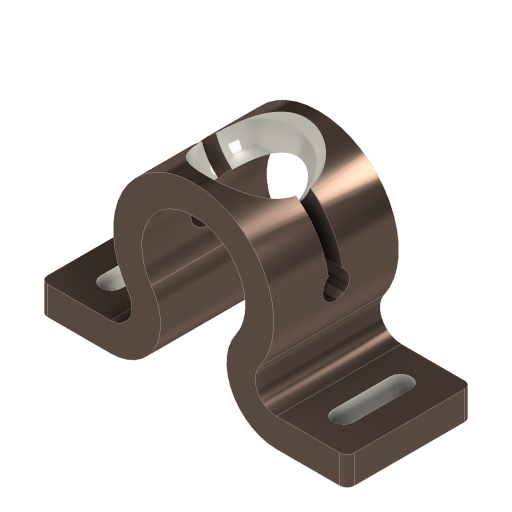
# Autodesk Inventor part: Part013. Fulcrum
Saved by Autodesk Inventor 2023.2 (Build 272271030, 271C)
## iProperties
Created: 2023-09-13
Part Number: Part013. Fulcrum
Material: Steel, Carbon
Document SubType Name: Modeling
Designer: User
Mass: 2408.89 g
Surface Area: 598.145 cm^2
Volume: 306.865 cm^3
Density: 7.85 g/cm^3
Appearance: Gunmetal - Antique Polished
Author: User
Autodesk Inventor part; units mm, degrees
ref_plane "YZ Plane" through (0, 0, 0) normal (1, 0, 0) x (0, 1, 0)
ref_plane "XZ Plane" through (0, 0, 0) normal (0, 1, 0) x (-1, 0, 0)
ref_plane "XY Plane" through (0, 0, 0) normal (0, 0, 1) x (1, 0, 0)
sketch "Sketch1" plane through (0, 0, 0) normal (0, 0, 1) x (1, 0, 0)
  line L0 (-86, -45) -> (-46.4758, -45)
  arc A0 (-46.4758, -45) -> (-36.6914, -26.0526) centre (-46.4758, -33) ccw
  arc A1 (36.6914, -26.0526) -> (-36.6914, -26.0526) centre (0, 0) ccw
  arc A2 (36.6914, -26.0526) -> (46.4758, -45) centre (46.4758, -33) ccw
  line L1 (46.4758, -45) -> (86, -45)
  line L2 (0, -90.5431) -> (0, 67.5905) construction
  line L3 (-86, -61) -> (-46.4758, -61)
  arc A3 (-46.4758, -61) -> (-23.6456, -16.7895) centre (-46.4758, -33) ccw
  arc A4 (23.6456, -16.7895) -> (-23.6456, -16.7895) centre (0, 0) ccw
  arc A5 (23.6456, -16.7895) -> (46.4758, -61) centre (46.4758, -33) ccw
  line L4 (46.4758, -61) -> (86, -61)
  line L5 (-86, -45) -> (-86, -61)
  line L6 (86, -45) -> (86, -61)
  dimension "d0" = 90
  dimension "d1" = 12
  dimension "d2" = 45
  dimension "d3" = 172
  dimension "d4" = 16
  constraints: 12 end point, 12 point on circle, 6 centre point, 3 tangent, 2 horizontal, 1 coincident, 1 parallel, 1 symmetric about line, 1 vertical, 6 other
  measures "d0" diameter of A1
  measures "d1" radius of A0
  measures "d2" distance from line of L0 point (0, 0)
  measures "d3" distance of L1.end L0.start
  measures "d4" radial gap between concentric circles of A1 A4
extrude "Extrusion1" add sketch "Sketch1" along normal mid plane 70
sketch "Sketch2" plane through (0, 0, 0) normal (1, 0, 0) x (0, 1, 0)
  arc A0 (6.3443, 4) -> (6.3443, -4) centre (0, 0) ccw
  line L0 (6.3443, 4) -> (45, 4)
  line L1 (45, 4) -> (45, -4)
  line L2 (45, -4) -> (6.3443, -4)
  line L3 (45, -35) -> (45, 35) projected
  dimension "d7" = 15
  dimension "d8" = 8
  constraints: 6 end point, 2 parallel, 2 point on circle, 1 centre point, 1 coincident, 1 collinear, 1 horizontal, 1 perpendicular
  measures "d7" diameter of A0
  measures "d8" distance between parallel lines of L2 L0
extrude "Extrusion2" cut sketch "Sketch2" along normal through all both and the other way through all
sketch "Sketch3" plane through (0, 0, 0) normal (0, 0, 1) x (1, 0, 0)
  arc A0 (0, 73) -> (0, 17) centre (0, 45) ccw
  line L0 (-86, -61) -> (-46.4758, -61) projected
  line L1 (0, 73) -> (0, 17)
  arc A1 (44.5505, 6.3443) -> (-44.5505, 6.3443) centre (0, 0) ccw projected
  point P0 (-66.2379, -61)
  point P1 (0, 45)
  dimension "d11" = 28
  dimension "d12" = 106
  constraints: 3 point on circle, 2 end point, 2 midpoint, 1 centre point, 1 vertical alignment
  measures "d11" radius of A0
  measures "d12" vertical distance of point (-66.238, -61) A0.centre
revolve "Revolution1" cut sketch "Sketch3" angle 360 about axis through (0, 73, 0) along (0, -1, 0)
sketch "Sketch4" plane through (46.4758, -45, 35) normal (0, 1, 0) x (1, 0, 0)
  line L0 (18.5242, 19) -> (18.5242, 51) construction
  line L1 (12.5242, 19) -> (12.5242, 51)
  line L2 (24.5242, 51) -> (24.5242, 19)
  arc A0 (12.5242, 19) -> (24.5242, 19) centre (18.5242, 19) ccw
  arc A1 (24.5242, 51) -> (12.5242, 51) centre (18.5242, 51) ccw
  point P0 (-46.4758, 35)
  point P1 (18.5242, 35)
  dimension "d14" = 6
  dimension "d15" = 32
  dimension "d16" = 65
  constraints: 8 end point, 4 point on circle, 4 tangent, 2 centre point, 1 horizontal alignment, 1 midpoint, 1 parallel, 1 vertical
  measures "d14" radius of A1
  measures "d15" distance of L2.start L2.end
  measures "d16" distance of point (-46.476, 35) point (18.524, 35)
extrude "Extrusion3" cut sketch "Sketch4" against normal through all
mirror "Mirror1" about plane through (0, 0, 0) normal (1, 0, 0) of "Extrusion3"
fillet "Fillet1" radius 4 4 edges at (-86, -53, 35) (-86, -53, -35) (86, -53, 35) (86, -53, -35)
body "Solid1"
